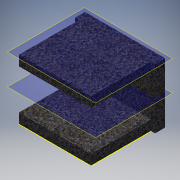
# Autodesk Inventor part: BaseMini
Saved by Autodesk Inventor 2016 (Build 200138000, 138)
## iProperties
Created: 2015-08-01
Part Number: BaseMini
Material: Concrete
Document SubType Name: Modeling
Designer: myhome
Density: 2.40731 g/cm^3
Appearance: Exposed Aggregate - Coarse
Mass: 40442.8 g
Surface Area: 8020 cm^2
Volume: 16800 cm^3
Author: myhome
Autodesk Inventor part; units mm, degrees
ref_plane "YZ Plane" through (0, 0, 0) normal (1, 0, 0) x (0, 1, 0)
ref_plane "XZ Plane" through (0, 0, 0) normal (0, 1, 0) x (-1, 0, 0)
ref_plane "XY Plane" through (0, 0, 0) normal (0, 0, 1) x (1, 0, 0)
sketch "Sketch1" plane through (0, 0, 0) normal (0, 0, 1) x (1, 0, 0)
  line L0 (0, 0) -> (400, 0)
  line L1 (400, 0) -> (400, 300)
  line L2 (400, 300) -> (0, 300)
  line L3 (0, 300) -> (0, 0)
  dimension "d0" = 400
  dimension "d1" = 300
  constraints: 8 end point, 2 parallel, 1 horizontal, 1 perpendicular
  measures "d0" distance of L1.end L2.end
  measures "d1" distance of L0.end L1.end
extrude "Extrusion1" add sketch "Sketch1" along normal blind 50
sketch "Sketch2" plane through (0, 0, 0) normal (0, 1, 0) x (-1, 0, 0)
  line L0 (0, 50) -> (-400, 50) projected
  line L1 (0, 50) -> (-20, 50)
  line L2 (-20, 50) -> (-20, 350)
  line L3 (-20, 350) -> (-380, 350)
  line L4 (-380, 350) -> (-380, 50)
  point P0 (0, 0)
  dimension "d4" = 20
  dimension "d5" = 300
  dimension "d6" = 360
  constraints: 8 end point, 3 perpendicular, 2 point on line
  measures "d4" distance of L0.start L1.end
  measures "d5" distance of L1.end L2.end
  measures "d6" distance of L2.end L3.end
sketch "Sketch3" plane through (0, 0, 0) normal (0, 1, 0) x (-1, 0, 0)
  line L0 (-20, 50) -> (-20, 350) projected
  line L1 (-20, 350) -> (-380, 350) projected
  line L2 (-380, 350) -> (-380, 50) projected
  point P0 (0, 0)
extrude "Extrusion2" add sketch "Sketch2" along normal blind 50
ref_plane "Work Plane1" through (0, 150, 0) normal (0, -1, 0) x (1, 0, 0)
ref_plane "Work Plane2" through (0, 300, 0) normal (0, -1, 0) x (1, 0, 0)
sketch "Sketch4" plane through (0, 300, 0) normal (0, -1, 0) x (1, 0, 0)
  line L0 (20, 350) -> (380, 350) projected
  line L1 (380, 350) -> (380, 50) projected
  line L2 (20, 50) -> (20, 350) projected
  line L3 (380, 50) -> (20, 50)
  line L4 (400, 50) -> (0, 50) projected
  point P0 (0, 0)
  constraints: 2 end point, 1 collinear
extrude "Extrusion3" add sketch "Sketch4" along normal blind 50
body "Solid1"
